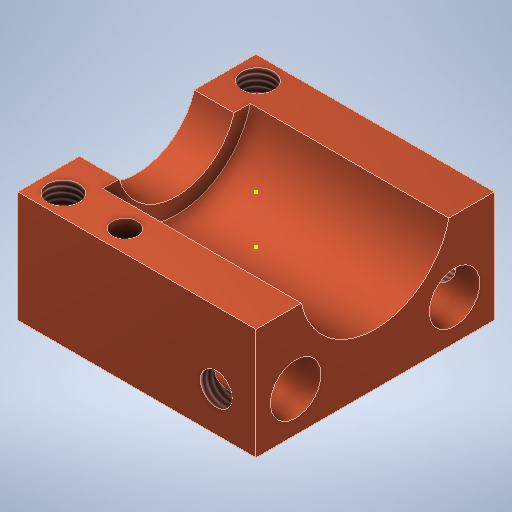
# Autodesk Inventor part: Rb oven housing top-back
Saved by Autodesk Inventor 2025.3 (Build 293356000, 356)
## iProperties
Created: 2025-04-11
Part Number: Rb oven housing top-back
Material: Copper
Document SubType Name: Modeling
Designer: Verðandi
Density: 8.94 g/cm^3
Appearance: Copper - Polished
Author: E. Moreno
Title: Carcasa Horno - Inferior
Autodesk Inventor part; units mm, degrees
ref_plane "YZ Plane" through (0, 0, 0) normal (1, 0, 0) x (0, 1, 0)
ref_plane "XZ Plane" through (0, 0, 0) normal (0, 1, 0) x (-1, 0, 0)
ref_plane "XY Plane" through (0, 0, 0) normal (0, 0, 1) x (1, 0, 0)
sketch "Sketch1" plane through (0, 0, 0) normal (0, 0, 1) x (1, 0, 0)
  line L0 (15, -7) -> (-15, -7)
  line L1 (-15, -7) -> (-15, 7)
  line L2 (-15, 7) -> (15, 7)
  line L3 (15, 7) -> (15, -7)
  line L4 (15, -7) -> (-15, 7) construction
  line L5 (-15, -7) -> (15, 7) construction
  point P0 (0, 0)
  dimension "d0" = 30
  dimension "d1" = 14
  constraints: 12 end point, 2 midpoint, 2 parallel, 1 horizontal, 1 perpendicular
  measures "d0" distance of L1.end L2.end
  measures "d1" distance of L0.end L1.end
extrude "Extrusion1" add sketch "Sketch1" along normal blind 30
sketch "Sketch3" plane through (15, -7, 0) normal (1, 0, 0) x (0, 0, -1)
  line L0 (0, 0) -> (-30, 0) projected
  line L1 (-15, 0) -> (-15, -2)
  arc A0 (-5.7129, 0) -> (-24.2871, 0) centre (-15, -2) ccw
  point P0 (0, 7)
  dimension "d4" = 2
  dimension "d5" = 19
  constraints: 2 end point, 2 point on circle, 2 point on line, 1 centre point, 1 coincident, 1 midpoint, 1 vertical
  measures "d4" distance of L1.start L1.end
  measures "d5" diameter of A0
extrude "Extrusion2" cut sketch "Sketch3" against normal blind 25
sketch "Sketch6" plane through (-15, 7, 0) normal (0, 1, 0) x (1, 0, 0)
  point P0 (15, 0)
sketch "Sketch7" plane through (15, -7, 0) normal (1, 0, 0) x (0, 0, -1)
  line L0 (0, 14) -> (-30, 14) projected
  line L1 (-30, 14) -> (-25, 14)
  line L2 (-25, 14) -> (-25, 9)
  line L3 (0, 14) -> (0, 0) projected
  line L4 (0, 14) -> (-5, 14)
  line L5 (-5, 14) -> (-5, 9)
  circle A0 centre (-25, 9) radius 3.175
  circle A1 centre (-5, 9) radius 3.175
  point P0 (0, 7)
  dimension "d21" = 5
  dimension "d22" = 5
  dimension "d23" = 5
  dimension "d24" = 5
  dimension "d25" = 6.35
  dimension "d26" = 6.35
  constraints: 8 end point, 2 centre point, 2 coincident, 2 point on line, 1 perpendicular, 1 vertical
  measures "d21" distance of L0.end L1.end
  measures "d22" distance of L1.end L2.end
  measures "d23" distance of L0.start L4.end
  measures "d24" distance of L4.end L5.end
  measures "d25" diameter of A0
  measures "d26" diameter of A1
extrude "Extrusion4" cut sketch "Sketch7" against normal blind 15
move or copy body "Move Body1" bodies to move or copy 1 copy no translate (-20, 0, 0)
move or copy body "Move Body2" bodies to move or copy 1 copy no translate (-5, 0, 0)
sketch "Sketch8" plane through (0, 0, 0) normal (1, 0, 0) x (0, 1, 0)
  point P0 (0, 0)
sketch "Sketch9" plane through (-40, 7, 0) normal (0, 1, 0) x (1, 0, 0)
  line L0 (30, -30) -> (0, -30) projected
  line L1 (0, -30) -> (0, -27.25)
  line L2 (0, 0) -> (0, -30) projected
  line L3 (0, -27.25) -> (3, -27.25)
  circle A0 centre (3, -27.25) radius 2
  line L4 (0, 0) -> (0, -2.75)
  line L5 (0, -2.75) -> (3, -2.75)
  circle A1 centre (3, -2.75) radius 2
  point P0 (40, 0)
  dimension "d35" = 2.75
  dimension "d36" = 3
  dimension "d37" = 4
  dimension "d38" = 2.75
  dimension "d39" = 4
  dimension "d40" = 3
  constraints: 8 end point, 2 centre point, 2 coincident, 2 perpendicular, 2 point on line
  measures "d35" distance of L0.end L1.end
  measures "d36" distance of L1.end L3.end
  measures "d37" diameter of A0
  measures "d38" distance of L2.start L4.end
  measures "d39" diameter of A1
  measures "d40" distance of L4.end L5.end
extrude "Extrusion5" cut sketch "Sketch9" against normal blind 14
sketch "Sketch14" plane through (-40, 7, 30) normal (0, 0, 1) x (1, 0, 0)
  line L0 (30, 0) -> (0, 0) projected
  line L1 (30, 0) -> (25, 0)
  line L2 (25, 0) -> (25, -5)
  circle A0 centre (25, -5) radius 2
  point P0 (40, -7)
  dimension "d47" = 5
  dimension "d48" = 5
  dimension "d49" = 4
  constraints: 4 end point, 1 centre point, 1 coincident, 1 perpendicular, 1 point on line
  measures "d47" distance of L0.start L1.end
  measures "d48" distance of L1.end L2.end
  measures "d49" diameter of A0
extrude "Extrusion6" cut sketch "Sketch14" against normal blind 3
sketch "Sketch15" plane through (-10, 7, 0) normal (0, 0, -1) x (-1, 0, 0)
  line L0 (0, -14) -> (0, 0) projected
  line L1 (0, 0) -> (5, 0)
  line L2 (0, 0) -> (30, 0) projected
  line L3 (5, 0) -> (5, -5)
  circle A0 centre (5, -5) radius 2
  point P0 (-10, -7)
  dimension "d52" = 5
  dimension "d53" = 5
  dimension "d54" = 4
  constraints: 4 end point, 1 centre point, 1 coincident, 1 perpendicular, 1 point on line
  measures "d52" distance of L0.end L1.end
  measures "d53" distance of L1.end L3.end
  measures "d54" diameter of A0
extrude "Extrusion7" cut sketch "Sketch15" against normal blind 4
thread "Thread3" size "M4x0.7" class "6H" standard "ANSI Metric M Profile" full length
thread "Thread4" size "M4x0.7" class "6H" standard "ANSI Metric M Profile" full length
sketch "Sketch16" plane through (-40, -7, 0) normal (-1, 0, 0) x (0, 0, 1)
  line L0 (0, 14) -> (30, 14) projected
  line L1 (0, 14) -> (15, 14)
  line L2 (15, 14) -> (15, -2)
  circle A0 centre (15, -2) radius 7.5
  point P0 (0, 7)
  dimension "d61" = 16
  dimension "d62" = 15
  constraints: 4 end point, 1 centre point, 1 coincident, 1 midpoint, 1 perpendicular
  measures "d61" distance of L1.end L2.end
  measures "d62" diameter of A0
extrude "Extrusion8" cut sketch "Sketch16" against normal blind 15
mirror "Mirror1" about plane through (0, 0, 0) normal (1, 0, 0) remove original yes
move or copy body "Move Body3" bodies to move or copy 1 copy no rotation origin (0, 0, 0) rotation axis (0, 1, 0) rotation angle 180 translate (20, 0, 60)
move or copy body "Move Body4" bodies to move or copy 1 copy no rotation origin (0, 0, 0) rotation axis (1, 0, 0) rotation angle -180 translate (0, 14, 120)
thread "Thread5" size "M4x0.7" class "6H" standard "ANSI Metric M Profile" full length
thread "Thread6" size "M4x0.7" class "6H" standard "ANSI Metric M Profile" full length
move or copy body "Move Body5" bodies to move or copy 1 copy no translate (20, 0, -70)
move or copy body "Move Body6" bodies to move or copy 1 copy no translate (-15, 0, 0)
move or copy body "Move Body7" bodies to move or copy 1 copy no translate (10, 0, -5)
move or copy body "Move Body8" bodies to move or copy 1 copy no translate (0, -8, 0)
move or copy body "Move Body9" bodies to move or copy 1 copy no translate (-10, 0, 0)
sketch "Sketch17" plane through (-15, 13, 15) normal (0, 1, 0) x (1, 0, 0)
  point P0 (15, 15)
sketch "Sketch18" plane through (-15, 13, 15) normal (0, 1, 0) x (1, 0, 0)
  line L0 (0, 0) -> (0, 2.75)
  line L1 (0, 7.7716) -> (0, 0) projected
  line L2 (0, 2.75) -> (10.75, 2.75)
  circle A0 centre (10.75, 2.75) radius 1.5875
  point P0 (15, 15)
  dimension "d87" = 2.75
  dimension "d88" = 10.75
  dimension "d89" = 3.175
  constraints: 4 end point, 1 centre point, 1 coincident, 1 perpendicular, 1 point on line
  measures "d87" distance of L0.start L0.end
  measures "d88" distance of L0.end L2.end
  measures "d89" diameter of A0
extrude "Extrusion9" cut sketch "Sketch18" against normal blind 10.5
equation "\"d55\" = d54"
body "Solid1"
